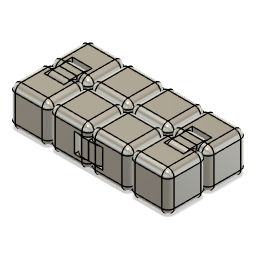
infinity_cube_rounded_and_scaled v28 (Autodesk Fusion 360 design; units mm, degrees)
Autodesk Fusion 360 part; units mm, degrees
note: some values were not read from the file. Chosen so that the rebuilt part matches the saved one: which bodies a step acts on; which face or edge a step refers to; which sketch regions a step uses.
sketch "BaseCubes" plane through (0, 0, 0) normal (0, 1, 0) x (1, 0, 0)
  line L0 (0, 0) -> (16, 0)
  line L1 (16, 0) -> (16, -16)
  line L2 (16, -16) -> (0, -16)
  line L3 (0, -16) -> (0, 0)
  line L4 (16.4, 0) -> (32.4, 0)
  line L5 (32.4, 0) -> (32.4, -16)
  line L6 (32.4, -16) -> (16.4, -16)
  line L7 (16.4, -16) -> (16.4, 0)
  dimension "d1" = 16
  dimension "d2" = 16
  dimension "d3" = 16
  dimension "d4" = 16
  dimension "d5" = 0.4
  constraint horizontal L0
  constraint vertical L1
  constraint horizontal L2
  constraint vertical L3
  constraint coincident L0.start L3.end
  constraint horizontal L4
  constraint vertical L5
  constraint horizontal L6
  constraint vertical L7
  constraint collinear L0 L4
  measures "d1" distance of L0.start L0.end
  measures "d2" distance of L0.start L2.end
  measures "d3" distance of L4.start L4.end
  measures "d4" distance of L4.start L6.end
  measures "d5" distance of L1 L7
extrude "Extrude1" add sketch "BaseCubes" along normal blind 16 contours L0 L1 L2 L3 makes body 1
extrude "Extrude2" add sketch "BaseCubes" along normal blind 16 separate body contours L4 L5 L6 L7 makes body 2
fillet "Fillet4" radius 2.5 5 faces at (21.7333, 16, 5.3333) (32.4, 5.3333, 5.3333) (27.0667, 5.3333, 16) (16.4, 10.6667, 10.6667) (21.7333, 10.6667, 0) on bodies 2
fillet "Fillet5" radius 2.5 6 faces at (5.3333, 16, 5.3333) (10.6667, 10.6667, 16) (16, 5.3333, 5.3333) (5.3333, 5.3333, 0) (5.3333, 0, 5.3333) (0, 10.6667, 10.6667) on bodies 1
sketch "Hinge1" plane through (0, 16, 0) normal (0, 1, 0) x (-1, 0, 0)
  line L0 (-4, 0) -> (-12, 0)
  line L1 (-12, 0) -> (-12, 5.6)
  line L2 (-12, 5.6) -> (-4, 5.6)
  line L3 (-4, 5.6) -> (-4, 0)
  line L4 (-4.4, 5.2) -> (-11.6, 5.2)
  line L5 (-11.6, 5.2) -> (-11.6, -0.24)
  line L6 (-11.6, -0.24) -> (-4.4, -0.24)
  line L7 (-4.4, -0.24) -> (-4.4, 5.2)
  line L8 (-13.5, 13.5) -> (-13.5, 2.5)
  line L9 (-13.5, 2.5) -> (-2.5, 2.5)
  line L10 (-2.5, 2.5) -> (-2.5, 13.5)
  line L11 (-2.5, 13.5) -> (-13.5, 13.5)
  dimension "d12" = 8
  dimension "d13" = 5.6
  dimension "d16" = 7.2
  dimension "d17" = 5.44
  dimension "d18" = 0.4
  dimension "d19" = 0.4
  constraint horizontal L0
  constraint vertical L1
  constraint horizontal L2
  constraint vertical L3
  constraint horizontal L4
  constraint vertical L5
  constraint horizontal L6
  constraint vertical L7
  measures "d12" distance of L0.start L0.end
  measures "d13" distance of L0.start L2.end
  measures "d16" distance of L4.start L4.end
  measures "d17" distance of L4.start L6.end
  measures "d18" distance of L3 L7
  measures "d19" distance of L2 L4
sketch "Hinge2" plane through (0, 0, 16) normal (0, 0, 1) x (1, 0, 0)
  line L0 (26.8, 12) -> (32.4, 12)
  line L1 (32.4, 12) -> (32.4, 4)
  line L2 (32.4, 4) -> (26.8, 4)
  line L3 (26.8, 4) -> (26.8, 12)
  line L4 (27.2, 11.6) -> (32.64, 11.6)
  line L5 (32.64, 11.6) -> (32.64, 4.4)
  line L6 (32.64, 4.4) -> (27.2, 4.4)
  line L7 (27.2, 4.4) -> (27.2, 11.6)
  line L8 (18.9, 2.5) -> (29.9, 2.5)
  line L9 (29.9, 2.5) -> (29.9, 13.5)
  line L10 (29.9, 13.5) -> (18.9, 13.5)
  line L11 (18.9, 13.5) -> (18.9, 2.5)
  dimension "d20" = 5.6
  dimension "d21" = 8
  dimension "d24" = 5.44
  dimension "d25" = 7.2
  dimension "d26" = 0.4
  dimension "d27" = 0.4
  constraint horizontal L0
  constraint vertical L1
  constraint horizontal L2
  constraint vertical L3
  constraint horizontal L4
  constraint vertical L5
  constraint horizontal L6
  constraint vertical L7
  measures "d20" distance of L0.start L0.end
  measures "d21" distance of L0.start L2.end
  measures "d24" distance of L4.start L4.end
  measures "d25" distance of L4.start L6.end
  measures "d26" distance of L3 L7
  measures "d27" distance of L0 L4
sketch "Hinge3" plane through (0, 0, 0) normal (0, -1, 0) x (1, 0, 0)
  line L0 (10.4, 12) -> (16, 12)
  line L1 (16, 12) -> (16, 4)
  line L2 (16, 4) -> (10.4, 4)
  line L3 (10.4, 4) -> (10.4, 12)
  line L4 (10.8, 11.6) -> (16.2, 11.6)
  line L5 (16.2, 11.6) -> (16.2, 4.4)
  line L6 (16.2, 4.4) -> (10.8, 4.4)
  line L7 (10.8, 4.4) -> (10.8, 11.6)
  line L8 (13.5, 13.5) -> (2.5, 13.5)
  line L9 (2.5, 13.5) -> (2.5, 2.5)
  line L10 (2.5, 2.5) -> (13.5, 2.5)
  line L11 (13.5, 2.5) -> (13.5, 13.5)
  dimension "d28" = 5.6
  dimension "d29" = 8
  dimension "d32" = 5.4
  dimension "d33" = 7.2
  dimension "d34" = 0.4
  dimension "d35" = 0.4
  constraint horizontal L0
  constraint vertical L1
  constraint horizontal L2
  constraint vertical L3
  constraint horizontal L4
  constraint vertical L5
  constraint horizontal L6
  constraint vertical L7
  measures "d28" distance of L0.start L0.end
  measures "d29" distance of L0.start L2.end
  measures "d32" distance of L4.start L4.end
  measures "d33" distance of L4.start L6.end
  measures "d34" distance of L0 L4
  measures "d35" distance of L3 L7
sketch "Hinge4" plane through (0, 0, 0) normal (0, -1, 0) x (1, 0, 0)
  line L0 (16.4, 12) -> (22, 12)
  line L1 (22, 12) -> (22, 4)
  line L2 (22, 4) -> (16.4, 4)
  line L3 (16.4, 4) -> (16.4, 12)
  line L4 (16.2, 11.6) -> (21.6, 11.6)
  line L5 (21.6, 11.6) -> (21.6, 4.4)
  line L6 (21.6, 4.4) -> (16.2, 4.4)
  line L7 (16.2, 4.4) -> (16.2, 11.6)
  line L8 (29.9, 13.5) -> (18.9, 13.5)
  line L9 (18.9, 13.5) -> (18.9, 2.5)
  line L10 (18.9, 2.5) -> (29.9, 2.5)
  line L11 (29.9, 2.5) -> (29.9, 13.5)
  dimension "d36" = 5.6
  dimension "d37" = 8
  dimension "d40" = 5.4
  dimension "d41" = 7.2
  dimension "d42" = 0.4
  dimension "d43" = 0.4
  constraint horizontal L0
  constraint vertical L1
  constraint horizontal L2
  constraint vertical L3
  constraint horizontal L4
  constraint vertical L5
  constraint horizontal L6
  constraint vertical L7
  measures "d36" distance of L0.start L0.end
  measures "d37" distance of L0.start L2.end
  measures "d40" distance of L4.start L4.end
  measures "d41" distance of L4.start L6.end
  measures "d42" distance of L0 L4
  measures "d43" distance of L1 L5
extrude "Extrude3" cut sketch "Hinge1" against normal blind 5.6 contours L0 L3 L7 L9 | L0 L5 L7 L9 | L1 L2 L3 L4 L5 L7 L9 | L0 L1 L5 L9 | L4 L5 L7 L9 bodies 1
extrude "Extrude4" add sketch "Hinge1" against normal blind 5.2 separate body contours L0 L5 L6 L7 | L0 L5 L7 L9 | L4 L5 L7 L9 makes body 3
extrude "Extrude5" cut sketch "Hinge2" against normal blind 5.6 contours L0 L2 L3 L4 L6 L7 L9 | L0 L1 L4 L9 | L4 L6 L7 L9 | L1 L4 L6 L9 | L1 L2 L6 L9 bodies 2
extrude "Extrude6" add sketch "Hinge2" against normal blind 5.2 separate body contours L4 L6 L7 L9 | L1 L4 L6 L9 | L1 L4 L5 L6 makes body 4
extrude "Extrude7" cut sketch "Hinge4" sketch "Hinge3" against normal blind 5.6 contours L0 L3 L4 L9 | L0 L1 L2 L4 L5 L6 L9 | L3 L4 L6 L9 | L4 L5 L6 L9 | L2 L3 L6 L9 of sketch 2 contours L0 L2 L3 L4 L6 L7 L11 | L0 L1 L4 L11 | L4 L6 L7 L11 | L1 L4 L6 L11 | L1 L2 L6 L11 bodies 1 2
extrude "Extrude8" add sketch "Hinge3" against normal blind 5.2 separate body contours L4 L6 L7 L11 | L1 L4 L6 L11 | L1 L4 L5 L6 makes body 5
extrude "Extrude9" add sketch "Hinge4" against normal blind 5.2 separate body contours L3 L4 L6 L9 | L3 L4 L6 L7 | L4 L5 L6 L9 makes body 6
fillet "Fillet1" radius 2.6 2 edges at (8, 16, 5.2) (8, 10.8, 5.2) on bodies 3
fillet "Fillet2" radius 2.6 2 edges at (27.2, 8, 10.8) (27.2, 8, 16) on bodies 4
fillet "Fillet3" radius 2.6 4 edges at (10.8, 5.2, 8) (10.8, 0, 8) (21.6, 5.2, 8) (21.6, 0, 8) on bodies 5 6
sketch "PinCube1" plane through (12, 0, 0) normal (-1, 0, 0) x (0, 0, 1)
  line L0 (0, 10.4) -> (5.6, 10.4)
  line L1 (5.6, 10.4) -> (5.6, 16)
  circle A0 centre (2.8, 13.2) radius 1
  circle A1 centre (2.8, 13.2) radius 1.25
  arc A2 (2.5, 16) -> (0, 13.5) centre (2.5, 13.5) ccw
  line L2 (0, 13.5) -> (0, 10.4)
  line L3 (5.6, 16) -> (2.5, 16)
  dimension "d64" = 2
  dimension "d65" = 2.5
  constraint concentric A0 A1
  measures "d64" diameter of A0
  measures "d65" diameter of A1
sketch "PinHinge1" plane through (4.4, 0, 0) normal (-1, 0, 0) x (0, 0, 1)
  arc A0 (2.6, 10.8) -> (2.6, 16) centre (2.6, 13.4) ccw
  line L0 (-0.24, 16) -> (-0.24, 10.8)
  circle A1 centre (2.8, 13.2) radius 1
  circle A2 centre (2.8, 13.2) radius 1.25
  line L1 (2.6, 16) -> (-0.24, 16)
  line L2 (-0.24, 10.8) -> (2.6, 10.8)
  point P0 (2.8, 13.2)
  dimension "d68" = 2
  dimension "d69" = 2.5
  constraint coincident P0 A1.centre
  constraint concentric A1 A2
  measures "d68" diameter of A1
  measures "d69" diameter of A2
sketch "PinCube2" plane through (0, 4, 0) normal (0, 1, 0) x (-1, 0, 0)
  line L0 (-32.4, 13.5) -> (-32.4, 10.4)
  line L1 (-32.4, 10.4) -> (-26.8, 10.4)
  line L2 (-26.8, 10.4) -> (-26.8, 16)
  line L3 (-26.8, 16) -> (-29.9, 16)
  circle A0 centre (-29.6, 13.2) radius 1
  circle A1 centre (-29.6, 13.2) radius 1.25
  arc A2 (-29.9, 16) -> (-32.4, 13.5) centre (-29.9, 13.5) ccw
  dimension "d70" = 2
  dimension "d71" = 2.5
  dimension "d72" = 2.8
  dimension "d73" = 2.8
  constraint concentric A0 A1
  measures "d70" diameter of A0
  measures "d71" diameter of A1
  measures "d72" distance of L0 A0.centre
  measures "d73" distance of L3 A0.centre
sketch "PinHinge2" plane through (0, 11.6, 0) normal (0, 1, 0) x (-1, 0, 0)
  arc A0 (-29.8, 10.8) -> (-29.8, 16) centre (-29.8, 13.4) ccw
  line L0 (-32.64, 16) -> (-32.64, 10.8)
  circle A1 centre (-29.6, 13.2) radius 1.25
  circle A2 centre (-29.6, 13.2) radius 1
  line L1 (-29.8, 16) -> (-32.64, 16)
  line L2 (-32.64, 10.8) -> (-29.8, 10.8)
  point P0 (-29.6, 13.2)
  dimension "d74" = 2.5
  dimension "d75" = 2
  constraint coincident P0 A1.centre
  constraint concentric A1 A2
  measures "d74" diameter of A1
  measures "d75" diameter of A2
sketch "PinCube3" plane through (0, 0, 4) normal (0, 0, 1) x (1, 0, 0)
  line L0 (16, 2.5) -> (16, 5.6)
  line L1 (16, 5.6) -> (10.4, 5.6)
  line L2 (10.4, 5.6) -> (10.4, 0)
  line L3 (10.4, 0) -> (13.5, 0)
  circle A0 centre (13.2, 2.8) radius 1
  circle A1 centre (13.2, 2.8) radius 1.25
  arc A2 (13.5, 0) -> (16, 2.5) centre (13.5, 2.5) ccw
  dimension "d76" = 2
  dimension "d77" = 2.5
  dimension "d78" = 2.8
  dimension "d79" = 2.8
  constraint concentric A0 A1
  measures "d76" diameter of A0
  measures "d77" diameter of A1
  measures "d78" distance of L0 A0.centre
  measures "d79" distance of L3 A0.centre
sketch "PinHinge3" plane through (0, 0, 11.6) normal (0, 0, 1) x (1, 0, 0)
  arc A0 (13.4, 5.2) -> (13.4, 0) centre (13.4, 2.6) ccw
  line L0 (16.2, 0) -> (16.2, 5.2)
  circle A1 centre (13.2, 2.8) radius 1
  circle A2 centre (13.2, 2.8) radius 1.25
  line L1 (13.4, 0) -> (16.2, 0)
  line L2 (16.2, 5.2) -> (13.4, 5.2)
  point P0 (13.2, 2.8)
  dimension "d80" = 2
  dimension "d81" = 2.5
  constraint coincident P0 A1.centre
  measures "d80" diameter of A1
  measures "d81" diameter of A2
sketch "PinCube4" plane through (0, 0, 12) normal (0, 0, -1) x (-1, 0, 0)
  line L0 (-16.4, 5.6) -> (-22, 5.6)
  line L1 (-22, 5.6) -> (-22, 0)
  circle A0 centre (-19.2, 2.8) radius 1
  circle A1 centre (-19.2, 2.8) radius 1.25
  line L2 (-16.4, 2.5) -> (-16.4, 5.6)
  line L3 (-22, 0) -> (-18.9, 0)
  arc A2 (-18.9, 0) -> (-16.4, 2.5) centre (-18.9, 2.5) ccw
  dimension "d82" = 2
  dimension "d83" = 2.5
  constraint concentric A0 A1
  measures "d82" diameter of A0
  measures "d83" diameter of A1
sketch "PinHinge4" plane through (0, 0, 4.4) normal (0, 0, -1) x (-1, 0, 0)
  arc A0 (-19, 5.2) -> (-19, 0) centre (-19, 2.6) ccw
  line L0 (-16.2, 0) -> (-16.2, 5.2)
  circle A1 centre (-19.2, 2.8) radius 1
  circle A2 centre (-19.2, 2.8) radius 1.25
  line L1 (-19, 0) -> (-16.2, 0)
  line L2 (-16.2, 5.2) -> (-19, 5.2)
  point P0 (-19.2, 2.8)
  dimension "d86" = 2
  dimension "d87" = 2.5
  constraint coincident P0 A1.centre
  measures "d86" diameter of A1
  measures "d87" diameter of A2
extrude "Extrude10" cut sketch "PinCube1" along normal blind 2.4 draft -25 contours A0 | A1 bodies 3
extrude "Extrude11" add sketch "PinCube1" along normal blind 2.4 draft -30 contours A0 bodies 1
extrude "Extrude12" cut sketch "PinHinge1" along normal blind 2.4 draft -25 contours A1 | A2 bodies 1
extrude "Extrude13" add sketch "PinHinge1" along normal blind 2.4 draft -30 contours A1 bodies 3
extrude "Extrude14" cut sketch "PinHinge2" along normal blind 2.4 draft -25 contours A1 | A2 bodies 2
extrude "Extrude15" add sketch "PinHinge2" along normal blind 2.4 draft -30 contours A2 bodies 4
extrude "Extrude16" cut sketch "PinCube2" along normal blind 2.4 draft -25 contours A0 | A1 bodies 4
extrude "Extrude17" add sketch "PinCube2" along normal blind 2.4 draft -30 contours A0 bodies 2
extrude "Extrude18" cut sketch "PinCube4" along normal blind 2.4 draft -25 contours A0 | A1 bodies 6
extrude "Extrude19" add sketch "PinCube4" along normal blind 2.4 draft -30 contours A0 bodies 2
extrude "Extrude20" cut sketch "PinHinge4" along normal blind 2.4 draft -25 contours A1 | A2 bodies 2
extrude "Extrude21" add sketch "PinHinge4" along normal blind 2.4 draft -30 contours A1 bodies 6
extrude "Extrude22" cut sketch "PinCube3" along normal blind 2.4 draft -25 contours A0 | A1 bodies 5
extrude "Extrude23" add sketch "PinCube3" along normal blind 2.4 draft -30 contours A0 bodies 1
extrude "Extrude24" cut sketch "PinHinge3" along normal blind 2.4 draft -25 contours A1 | A2 bodies 1
extrude "Extrude25" add sketch "PinHinge3" along normal blind 2.4 draft -30 contours A1 bodies 5
ref_plane "WorkPlane1" through (24.4, 8, -0.2) normal (0, 0, -1) x (-1, 0, 0)
ref_plane "WorkPlane2" through (32.6, 8, 8) normal (1, 0, 0) x (0, 0, -1)
mirror "Mirror1" about plane through (24.4, 8, -0.2) normal (0, 0, -1) of bodies 1 3 5 makes body 7 at (0, 9.8333, -6.5667) makes body 8 at (6.8, 12.5333, -0.16) makes body 9 at (16.2, 1.7333, -9.6)
mirror "Mirror2" about plane through (32.6, 8, 8) normal (1, 0, 0) of bodies 2 4 6 makes body 10 at (32.56, 9.2, 14.2667) makes body 11 at (49, 3.4667, 9.2) makes body 12 at (42.6333, 16, 6.1667)
mirror "Mirror4" about plane through (24.4, 8, -0.2) normal (0, 0, -1) of bodies 2 12 11 10 4 6 makes body 13 at (26.2333, 9.8333, -0.4) makes body 14 at (32.64, 9.2, -14.6667) makes body 15 at (16.2, 3.4667, -9.6) makes body 16 at (32.56, 9.2, -14.6667) makes body 17 at (49, 3.4667, -9.6) makes body 18 at (42.6333, 16, -6.5667)
copy_body "CopyPasteBodies1" bodies 1 3 5 7 8 9 makes body 19 makes body 20 makes body 21 makes body 22 makes body 23 makes body 24
move_body "Move1" bodies 19 20 21 22 23 24 to x (-1, 0, 0) y (0, 1, 0) z (0, 0, -1) at (0, 0, 0)
move_body "Move2" bodies 19 20 21 22 23 24 to x (1, 0, 0) y (0, 1, 0) z (0, 0, 1) at (65.2, 0, -0.4)
named bodies: "Cube1", "Cube2", "Cube3", "Cube7", "Cube8", "Cube4", "Cube5", "Cube6"
